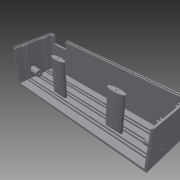
# Autodesk Inventor part: Krabicka_dolna_cast
Saved by Autodesk Inventor 2014 (Build 180170000, 170)
## iProperties
Created: 2017-08-29
Part Number: Krabicka_dolna_cast
Material: Všeobecné
Document SubType Name: Modeling
Designer: N
Density: 1 g/cm^3
Appearance: Výchozí
Author: N
Autodesk Inventor part; units mm, degrees
ref_plane "YZ Plane" through (0, 0, 0) normal (1, 0, 0) x (0, 1, 0)
ref_plane "XZ Plane" through (0, 0, 0) normal (0, 1, 0) x (-1, 0, 0)
ref_plane "XY Plane" through (0, 0, 0) normal (0, 0, 1) x (1, 0, 0)
sketch "Náčrt12" plane through (0, 0, 0) normal (0, 1, 0) x (-1, 0, 0)
  line L0 (0, 0) -> (177.8, 0)
  line L1 (177.8, 0) -> (177.8, 50.8)
  line L2 (177.8, 50.8) -> (0, 50.8)
  line L3 (0, 50.8) -> (0, 0)
  dimension "d34" = 50.8
  dimension "d35" = 177.8
  constraints: 8 end point, 2 parallel, 1 horizontal, 1 perpendicular
  measures "d34" distance between parallel lines of L0 L2
  measures "d35" distance between parallel lines of L1 L3
extrude "Vysunutí10" add sketch "Náčrt12" along normal blind 2.54
sketch "Náčrt13" plane through (0, 0, 0) normal (0, -1, 0) x (1, 0, 0)
  line L0 (0, 50.8) -> (0, 0) projected
  line L1 (-177.8, 50.8) -> (0, 50.8) projected
  line L2 (-177.8, 0) -> (-177.8, 50.8) projected
  line L3 (0, 0) -> (-177.8, 0) projected
  line L4 (-175.26, 0) -> (-175.26, 48.26)
  line L5 (-175.26, 48.26) -> (-2.54, 48.26)
  line L6 (-2.54, 48.26) -> (-2.54, 0)
  line L7 (-175.26, 10.16) -> (-2.54, 10.16)
  line L8 (-2.54, 10.16) -> (-2.54, 7.62)
  line L9 (-2.54, 7.62) -> (-175.26, 7.62)
  line L10 (-175.26, 7.62) -> (-175.26, 10.16)
  line L11 (-175.26, 22.86) -> (-2.54, 22.86)
  line L12 (-2.54, 22.86) -> (-2.54, 20.32)
  line L13 (-2.54, 20.32) -> (-175.26, 20.32)
  line L14 (-175.26, 20.32) -> (-175.26, 22.86)
  line L15 (-175.26, 35.56) -> (-2.54, 35.56)
  line L16 (-2.54, 35.56) -> (-2.54, 33.02)
  line L17 (-2.54, 33.02) -> (-175.26, 33.02)
  line L18 (-175.26, 33.02) -> (-175.26, 35.56)
  line L19 (-175.26, 40.64) -> (-2.54, 40.64)
  line L20 (-2.54, 40.64) -> (-2.54, 38.1)
  line L21 (-2.54, 38.1) -> (-175.26, 38.1)
  line L22 (-175.26, 38.1) -> (-175.26, 40.64)
  line L23 (-175.26, 15.24) -> (-2.54, 15.24)
  line L24 (-2.54, 15.24) -> (-2.54, 12.7)
  line L25 (-2.54, 12.7) -> (-175.26, 12.7)
  line L26 (-175.26, 12.7) -> (-175.26, 15.24)
  line L27 (-175.26, 27.94) -> (-2.54, 27.94)
  line L28 (-2.54, 27.94) -> (-2.54, 25.4)
  line L29 (-2.54, 25.4) -> (-175.26, 25.4)
  line L30 (-175.26, 25.4) -> (-175.26, 27.94)
  dimension "d73" = 2.54
  constraints: 54 end point, 14 point on line, 13 parallel, 8 perpendicular, 6 horizontal
  measures "d73" distance between parallel lines of L1 L5
extrude "Vysunutí11" add sketch "Náčrt13" along normal blind 43.18 contours L0 L3 L6 L5 L4 L2 L1
sketch "Náčrt14" plane through (0, 0, 0) normal (0, -1, 0) x (1, 0, 0)
  line L0 (-2.54, 0) -> (-2.54, 48.26) projected
  line L1 (-175.26, 48.26) -> (-175.26, 0) projected
  line L2 (-2.54, 0) -> (-175.26, 0) projected
  line L3 (-175.26, 9.525) -> (-2.54, 9.525)
  line L4 (-2.54, 9.525) -> (-2.54, 11.43)
  line L5 (-2.54, 11.43) -> (-175.26, 11.43)
  line L6 (-175.26, 11.43) -> (-175.26, 9.525)
  line L7 (-175.26, 15.24) -> (-2.54, 15.24)
  line L8 (-2.54, 15.24) -> (-2.54, 13.335)
  line L9 (-2.54, 13.335) -> (-175.26, 13.335)
  line L10 (-175.26, 13.335) -> (-175.26, 15.24)
  line L11 (-175.26, 24.13) -> (-2.54, 24.13)
  line L12 (-2.54, 24.13) -> (-2.54, 22.225)
  line L13 (-2.54, 22.225) -> (-175.26, 22.225)
  line L14 (-175.26, 22.225) -> (-175.26, 24.13)
  line L15 (-175.26, 27.94) -> (-2.54, 27.94)
  line L16 (-2.54, 27.94) -> (-2.54, 26.035)
  line L17 (-2.54, 26.035) -> (-175.26, 26.035)
  line L18 (-175.26, 26.035) -> (-175.26, 27.94)
  line L19 (-175.26, 40.64) -> (-2.54, 40.64)
  line L20 (-2.54, 40.64) -> (-2.54, 38.735)
  line L21 (-2.54, 38.735) -> (-175.26, 38.735)
  line L22 (-175.26, 38.735) -> (-175.26, 40.64)
  line L23 (-175.26, 36.83) -> (-2.54, 36.83)
  line L24 (-2.54, 36.83) -> (-2.54, 34.925)
  line L25 (-2.54, 34.925) -> (-175.26, 34.925)
  line L26 (-175.26, 34.925) -> (-175.26, 36.83)
  point P0 (0, 0)
  dimension "d59" = 11.43
  dimension "d60" = 1.905
  dimension "d61" = 1.905
  dimension "d62" = 1.905
  dimension "d63" = 1.905
  dimension "d64" = 1.905
  dimension "d65" = 1.905
  dimension "d66" = 1.905
  dimension "d67" = 10.795
  dimension "d68" = 1.905
  dimension "d69" = 10.795
  dimension "d70" = 1.905
  constraints: 48 end point, 12 parallel, 11 point on line, 6 horizontal, 6 perpendicular, 1 midpoint
  measures "d59" distance between parallel lines of L2 L5
  measures "d60" distance between parallel lines of L5 L3
  measures "d61" distance between parallel lines of L7 L9
  measures "d62" distance between parallel lines of L5 L9
  measures "d63" distance between parallel lines of L13 L11
  measures "d64" distance between parallel lines of L17 L15
  measures "d65" distance between parallel lines of L23 L25
  measures "d66" distance between parallel lines of L19 L21
  measures "d67" distance between parallel lines of L11 L9
  measures "d68" distance between parallel lines of L17 L11
  measures "d69" distance between parallel lines of L23 L17
  measures "d70" distance between parallel lines of L21 L23
extrude "Vysunutí12" add sketch "Náčrt14" along normal blind 1.905 contours L3 L1 L5 L0 | L9 L1 L7 L0 | L13 L1 L11 L0 | L17 L1 L15 L0 | L25 L1 L23 L0 | L21 L1 L19 L0
sketch "Náčrt16" plane through (0, -1.905, 0) normal (0, -1, 0) x (1, 0, 0)
  line L0 (-2.54, 9.525) -> (-175.26, 9.525) projected
  line L1 (-175.26, 11.43) -> (-173.3563, 11.43)
  line L2 (-173.3563, 11.43) -> (-173.3563, 9.525)
  line L3 (-173.3563, 9.525) -> (-175.26, 9.525)
  line L4 (-175.26, 9.525) -> (-175.26, 11.43)
  line L5 (-2.54, 11.43) -> (-4.435, 11.43)
  line L6 (-4.435, 11.43) -> (-4.435, 9.525)
  line L7 (-4.435, 9.525) -> (-2.54, 9.525)
  line L8 (-2.54, 9.525) -> (-2.54, 11.43)
  point P0 (0, 0)
  constraints: 16 end point, 4 parallel, 2 horizontal, 2 perpendicular, 2 point on line
extrude "Vysunutí13" add sketch "Náčrt16" along normal up to surface (41.275 mm away)
sketch "Náčrt17" plane through (0, -1.905, 0) normal (0, -1, 0) x (1, 0, 0)
  line L0 (-2.54, 13.335) -> (-175.26, 13.335) projected
  line L1 (-175.26, 15.24) -> (-173.3476, 15.24)
  line L2 (-173.3476, 15.24) -> (-173.3476, 13.335)
  line L3 (-173.3476, 13.335) -> (-175.26, 13.335)
  line L4 (-175.26, 13.335) -> (-175.26, 15.24)
  line L5 (-2.54, 15.24) -> (-4.4371, 15.24)
  line L6 (-4.4371, 15.24) -> (-4.4371, 13.335)
  line L7 (-4.4371, 13.335) -> (-2.54, 13.335)
  line L8 (-2.54, 13.335) -> (-2.54, 15.24)
  point P0 (0, 0)
  constraints: 16 end point, 4 parallel, 2 horizontal, 2 perpendicular, 2 point on line
extrude "Vysunutí14" add sketch "Náčrt17" along normal up to surface (41.275 mm away)
sketch "Náčrt18" plane through (0, -1.905, 0) normal (0, -1, 0) x (1, 0, 0)
  line L0 (-175.26, 34.925) -> (-175.26, 36.83) projected
  line L1 (-175.26, 34.925) -> (-2.54, 34.925) projected
  line L2 (-175.26, 36.83) -> (-173.3455, 36.83)
  line L3 (-173.3455, 36.83) -> (-173.3455, 34.925)
  line L4 (-173.3455, 34.925) -> (-175.26, 34.925)
  line L5 (-175.26, 34.925) -> (-175.26, 36.83)
  line L6 (-2.54, 36.83) -> (-4.4393, 36.83)
  line L7 (-4.4393, 36.83) -> (-4.4393, 34.925)
  line L8 (-4.4393, 34.925) -> (-2.54, 34.925)
  line L9 (-2.54, 34.925) -> (-2.54, 36.83)
  point P0 (0, 0)
  constraints: 16 end point, 4 parallel, 2 horizontal, 2 perpendicular, 2 point on line
extrude "Vysunutí15" add sketch "Náčrt18" along normal up to surface (41.275 mm away)
sketch "Náčrt19" plane through (0, -1.905, 0) normal (0, -1, 0) x (1, 0, 0)
  line L0 (-175.26, 38.735) -> (-175.26, 40.64) projected
  line L1 (-2.54, 38.735) -> (-175.26, 38.735) projected
  line L2 (-175.26, 40.64) -> (-173.3529, 40.64)
  line L3 (-173.3529, 40.64) -> (-173.3529, 38.735)
  line L4 (-173.3529, 38.735) -> (-175.26, 38.735)
  line L5 (-175.26, 38.735) -> (-175.26, 40.64)
  line L6 (-2.54, 40.64) -> (-4.4393, 40.64)
  line L7 (-4.4393, 40.64) -> (-4.4393, 38.735)
  line L8 (-4.4393, 38.735) -> (-2.54, 38.735)
  line L9 (-2.54, 38.735) -> (-2.54, 40.64)
  point P0 (0, 0)
  constraints: 16 end point, 4 parallel, 2 horizontal, 2 perpendicular, 2 point on line
extrude "Vysunutí16" add sketch "Náčrt19" along normal up to surface (41.275 mm away)
sketch "Náčrt20" plane through (0, -43.18, 0) normal (0, -1, 0) x (1, 0, 0)
  line L0 (-175.26, 40.64) -> (-175.26, 48.26) projected
  line L1 (0, 50.8) -> (-177.8, 50.8) projected
  line L2 (-170.18, 50.8) -> (-149.86, 50.8)
  line L3 (-149.86, 50.8) -> (-149.86, 48.26)
  line L4 (-149.86, 48.26) -> (-170.18, 48.26)
  line L5 (-170.18, 48.26) -> (-170.18, 50.8)
  dimension "d83" = 20.32
  dimension "d84" = 25.4
  constraints: 8 end point, 2 parallel, 1 horizontal, 1 perpendicular, 1 point on line
  measures "d83" distance between parallel lines of L5 L3
  measures "d84" distance between parallel lines of L0 L3
extrude "Vysunutí17" cut sketch "Náčrt20" against normal blind 9.525
sketch "Náčrt21" plane through (0, 0, 0) normal (0, -1, 0) x (1, 0, 0)
  line L0 (-175.26, 15.24) -> (-2.54, 15.24) projected
  line L1 (-2.54, 13.335) -> (-175.26, 13.335) projected
  line L2 (-2.54, 24.13) -> (-175.26, 24.13) projected
  ellipse E0 centre (-127, 18.7502) end of major axis (-116.84, 18.7502) minor radius 3.175
  ellipse E1 centre (-50.8, 18.7502) end of major axis (-40.64, 18.7502) minor radius 3.175
  line L3 (-2.54, 0) -> (-175.26, 0) projected
  line L4 (-175.26, 22.225) -> (-175.26, 15.24) projected
  point P0 (0, 0)
  dimension "d92" = 10.16
  dimension "d93" = 10.16
  dimension "d122" = 3.175
  dimension "d120" = 18.7502
  dimension "d121" = 48.26
  dimension "d123" = 76.2
  constraints: 2 horizontal, 4 other
  measures "d120" distance from line of L3 point (-127, 18.75)
  measures "d121" distance from line of L4 point (-127, 18.75)
  measures "d123" distance of point (-50.8, 18.75) point (-127, 18.75)
extrude "Vysunutí18" add sketch "Náčrt21" along normal up to surface (43.18 mm away)
sketch "Náčrt22" plane through (-127, -43.18, 18.7502) normal (0, -1, 0) x (1, 0, 0)
  ellipse E0 centre (0, 0) end of major axis (-10.16, 0) minor radius 3.175 projected
  circle A0 centre (0, 0) radius 0.9525
  point P0 (127, -18.7502)
  dimension "d96" = 1.905
  constraints: 1 centre point, 1 coincident, 1 other
  measures "d96" diameter of A0
extrude "Vysunutí19" cut sketch "Náčrt22" against normal blind 20.32 contours A0
sketch "Náčrt23" plane through (-50.8, -43.18, 18.7502) normal (0, -1, 0) x (1, 0, 0)
  ellipse E0 centre (0, 0) end of major axis (-10.16, 0) minor radius 3.175 projected
  circle A0 centre (0, 0) radius 0.9525
  point P0 (50.8, -18.7502)
  dimension "d99" = 1.905
  constraints: 1 centre point, 1 coincident, 1 other
  measures "d99" diameter of A0
extrude "Vysunutí20" cut sketch "Náčrt23" against normal blind 20.32 contours A0
sketch "Náčrt24" plane through (0, -43.18, 0) normal (0, -1, 0) x (1, 0, 0)
  line L0 (-149.86, 50.8) -> (-149.86, 48.26) projected
  line L1 (-2.54, 48.26) -> (-2.54, 40.64) projected
  line L2 (-2.54, 0) -> (0, 0) projected
  line L3 (0, 0) -> (0, 50.8) projected
  line L4 (0, 50.8) -> (-149.86, 50.8) projected
  line L5 (-1.27, 0) -> (-1.27, 49.53)
  line L6 (-1.27, 49.53) -> (-149.86, 49.53)
  constraints: 4 end point, 2 midpoint, 1 parallel
extrude "Vysunutí21" add sketch "Náčrt24" along normal blind 1.27
sketch "Náčrt25" plane through (0, -43.18, 0) normal (0, -1, 0) x (1, 0, 0)
  line L0 (-170.18, 48.26) -> (-170.18, 50.8) projected
  line L1 (-170.18, 50.8) -> (-177.8, 50.8) projected
  line L2 (-177.8, 50.8) -> (-177.8, 0) projected
  line L3 (-177.8, 0) -> (-175.26, 0) projected
  line L4 (-175.26, 48.26) -> (-170.18, 48.26) projected
  line L5 (-176.53, 0) -> (-176.53, 49.53)
  line L6 (-176.53, 49.53) -> (-170.18, 49.53)
  point P0 (0, 0)
  constraints: 4 end point, 2 midpoint, 1 perpendicular
extrude "Vysunutí22" add sketch "Náčrt25" along normal blind 1.27
sketch "Náčrt27" plane through (-2.54, 0, 27.94) normal (-1, 0, 0) x (0, 0, 1)
  circle A0 centre (-9.2075, -10.16) radius 4.445
  point P0 (-27.94, 0)
  dimension "d110" = 8.89
  constraints: 1 centre point
  measures "d110" diameter of A0
extrude "Vysunutí23" add sketch "Náčrt27" along normal blind 12.7
sketch "Náčrt28" plane through (-15.24, -10.16, 18.7325) normal (-1, 0, 0) x (0, 0, 1)
  circle A0 centre (0, 0) radius 4.445 projected
  circle A1 centre (0, 0) radius 0.9525
  point P0 (-18.7325, 10.16)
  dimension "d113" = 1.905
  constraints: 1 centre point, 1 coincident
  measures "d113" diameter of A1
extrude "Vysunutí24" cut sketch "Náčrt28" against normal through all contours A1
sketch "Náčrt30" plane through (-175.26, 0, 22.225) normal (1, 0, 0) x (0, 0, -1)
  circle A0 centre (3.4925, -10.16) radius 4.445 projected
  point P0 (22.225, 0)
extrude "Vysunutí25" add sketch "Náčrt30" along normal blind 12.7
sketch "Náčrt31" plane through (-162.56, -10.16, 18.7325) normal (1, 0, 0) x (0, 0, -1)
  circle A0 centre (0, 0) radius 0.9525 projected
  point P0 (18.7325, 10.16)
extrude "Vysunutí26" cut sketch "Náčrt31" against normal through all
